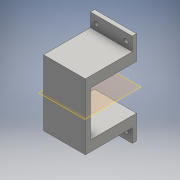
# Autodesk Inventor part: BaseClamp
Saved by Autodesk Inventor 2016 (Build 200138000, 138)
## iProperties
Created: 2017-11-27
Part Number: BaseClamp
Material: Generic
Document SubType Name: Modeling
Designer: alex
Density: 1 g/cm^3
Appearance: Default
Author: alex
Autodesk Inventor part; units mm, degrees
ref_plane "YZ Plane" through (0, 0, 0) normal (1, 0, 0) x (0, 1, 0)
ref_plane "XZ Plane" through (0, 0, 0) normal (0, 1, 0) x (-1, 0, 0)
sketch "Sketch1" plane through (0, 0, 0) normal (0, 1, 0) x (-1, 0, 0)
  line L0 (20, 31.455) -> (-20, 31.455)
  line L1 (-20, 31.455) -> (-20, -31.455)
  line L2 (-20, -31.455) -> (20, -31.455)
  line L3 (20, -31.455) -> (20, 31.455)
  point P0 (0, 0)
  point P1 (0, 31.455)
  point P2 (20, 0)
  dimension "d0" = 40
  dimension "d1" = 62.91
  constraints: 8 end point, 2 midpoint, 2 parallel, 1 horizontal, 1 horizontal alignment, 1 perpendicular, 1 vertical alignment
  measures "d0" distance of L0.start L0.end
  measures "d1" distance of L2.end L0.start
extrude "Extrusion1" add sketch "Sketch1" along normal blind 5
sketch "Sketch2" plane through (0, 5, 0) normal (0, 1, 0) x (1, 0, 0)
  line L0 (-20, -31.455) -> (20, -31.455) projected
  line L1 (20, -31.455) -> (20, 31.455) projected
  line L2 (-20, -31.455) -> (20, -31.455)
  line L3 (20, -31.455) -> (20, -21.455)
  line L4 (20, -21.455) -> (-20, -21.455)
  line L5 (-20, -21.455) -> (-20, -31.455)
  line L6 (-20, 31.4422) -> (20, 31.4422)
  line L7 (20, 31.4422) -> (20, 21.4422)
  line L8 (20, 21.4422) -> (-20, 21.4422)
  line L9 (-20, 21.4422) -> (-20, 31.4422)
  line L10 (20, 31.455) -> (-20, 31.455) projected
  point P0 (0, 0)
  dimension "d4" = 10
  dimension "d5" = 10
  dimension "d6" = 0.0128
  dimension "d7" = 40
  constraints: 16 end point, 4 parallel, 2 horizontal, 2 perpendicular, 2 point on line
  measures "d4" distance between parallel lines of L0 L4
  measures "d5" distance of L8.end L6.start
  measures "d6" distance between parallel lines of L10 L6
  measures "d7" distance between parallel lines of L9 L1
extrude "Extrusion2" add sketch "Sketch2" along normal blind 43.91
sketch "Sketch3" plane through (20, 5, -31.4422) normal (0, 0, -1) x (-1, 0, 0)
  line L0 (40, -5) -> (40, 43.91) projected
  line L1 (0, -5) -> (0, 43.91) projected
  line L2 (40, 43.91) -> (0, 43.91)
  line L3 (0, 43.91) -> (0, 39.91)
  line L4 (0, 39.91) -> (40, 39.91)
  line L5 (40, 39.91) -> (40, 43.91)
  point P0 (20, -5)
  dimension "d10" = 4
  constraints: 8 end point, 2 parallel, 1 horizontal, 1 perpendicular, 1 point on line
  measures "d10" distance between parallel lines of L2 L4
extrude "Extrusion3" add sketch "Sketch3" along normal blind 13
sketch "Sketch5" plane through (-20, 44.91, -31.4422) normal (0, -1, 0) x (1, 0, 0)
  circle A0 centre (34, -6.0128) radius 2
  circle A1 centre (6, -6.0128) radius 2
  line L0 (40, 0) -> (40, -13) projected
  line L1 (0, 0) -> (0, -13) projected
  line L2 (40, -0.0128) -> (0, -0.0128) projected
  point P0 (20, 31.4422)
  dimension "d17" = 4
  dimension "d18" = 4
  dimension "d19" = 6
  dimension "d20" = 6
  dimension "d21" = 6
  constraints: 2 centre point, 1 horizontal alignment
  measures "d17" diameter of A0
  measures "d18" diameter of A1
  measures "d19" distance from line of L0 A0.centre
  measures "d20" distance from line of L1 A1.centre
  measures "d21" distance from line of L2 A0.centre
extrude "Extrusion5" cut sketch "Sketch5" against normal through all
mirror "Mirror1" about plane through (0, 0, 0) normal (0, 0, 1) of "Extrusion3", "Extrusion5"
body "Solid1"
